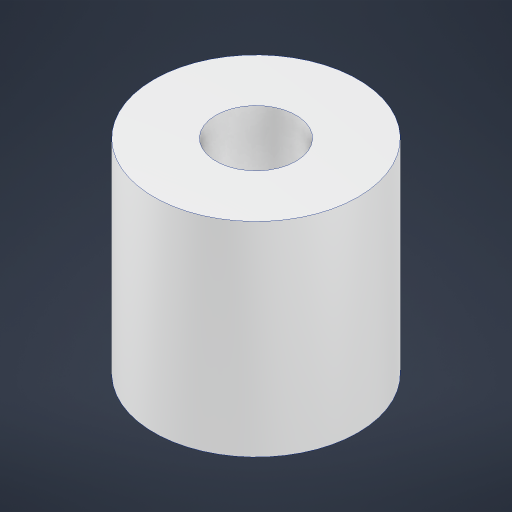
# Autodesk Inventor part: Standoff
Saved by Autodesk Inventor 2024.3 (Build 283343000, 343)
## iProperties
Created: 2024-12-08
Part Number: Standoff
Material: Aluminum 6061
Document SubType Name: Modeling
Designer: kaito
Density: 2.7 g/cm^3
Appearance: Aluminum - Flat
Author: kaito
Autodesk Inventor part; units mm, degrees
ref_plane "YZ Plane" through (0, 0, 0) normal (1, 0, 0) x (0, 1, 0)
ref_plane "XZ Plane" through (0, 0, 0) normal (0, 1, 0) x (-1, 0, 0)
ref_plane "XY Plane" through (0, 0, 0) normal (0, 0, 1) x (1, 0, 0)
sketch "Sketch1" plane through (0, 0, 0) normal (0, 1, 0) x (-1, 0, 0)
  circle A0 centre (0, 0) radius 6.35
  circle A1 centre (0, 0) radius 2.4892
  dimension "d0" = 12.7
  dimension "d1" = 4.9784
  constraints: 2 centre point, 2 coincident
  measures "d0" diameter of A0
  measures "d1" diameter of A1
extrude "Extrusion1" add sketch "Sketch1" along normal blind 12.7
body "Solid1"
